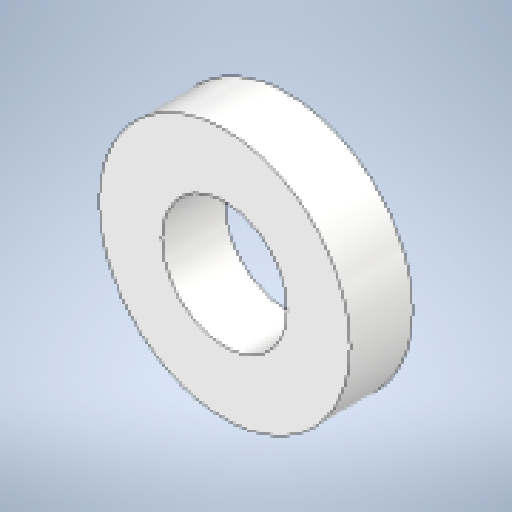
# Autodesk Inventor part: Spacer
Saved by Autodesk Inventor 2023.2 (Build 272271000, 271)
## iProperties
Created: 2024-01-21
Part Number: Spacer
Material: UHMW, White
Document SubType Name: Modeling
Designer: Nathan Cai
Density: 0.94 g/cm^3
Appearance: Smooth - White
Mass: 0.28355 g
Surface Area: 3.80031 cm^2
Volume: 0.301649 cm^3
Author: Nathan Cai
Autodesk Inventor part; units mm, degrees
ref_plane "YZ Plane" through (0, 0, 0) normal (1, 0, 0) x (0, 1, 0)
ref_plane "XZ Plane" through (0, 0, 0) normal (0, 1, 0) x (-1, 0, 0)
ref_plane "XY Plane" through (0, 0, 0) normal (0, 0, 1) x (1, 0, 0)
sketch "Sketch1" plane through (0, 0, 0) normal (0, 0, 1) x (1, 0, 0)
  circle A0 centre (0, 0) radius 3.175
  circle A1 centre (0, 0) radius 6.35
  dimension "d0" = 6.35
  dimension "d1" = 12.7
  constraints: 2 centre point, 2 coincident
  measures "d0" diameter of A0
  measures "d1" diameter of A1
extrude "Extrusion1" add sketch "Sketch1" along normal blind 3.175
body "Solid1"
